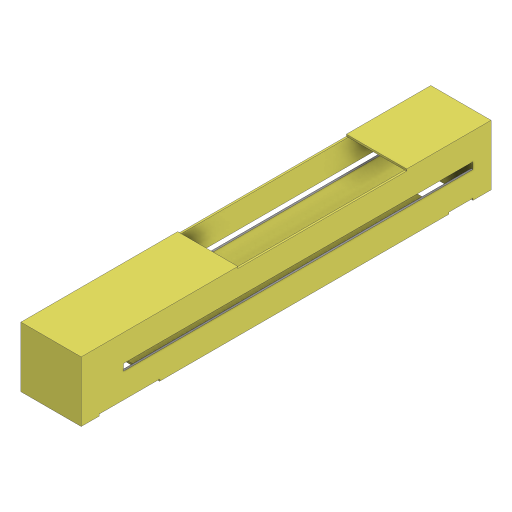
# Autodesk Inventor part: GUIA_CUADRADA
Saved by Autodesk Inventor 2024 (Build 280153000, 153)
## iProperties
Created: 2024-08-15
Part Number: GUIA_CUADRADA
Material: Generic
Document SubType Name: Modeling
Designer: Jhuliams
Density: 1 g/cm^3
Appearance: Default
Author: Jhuliams
Autodesk Inventor part; units mm, degrees
ref_plane "YZ Plane" through (0, 0, 0) normal (1, 0, 0) x (0, 1, 0)
ref_plane "XZ Plane" through (0, 0, 0) normal (0, 1, 0) x (-1, 0, 0)
ref_plane "XY Plane" through (0, 0, 0) normal (0, 0, 1) x (1, 0, 0)
sketch "Sketch1" plane through (0, 0, 0) normal (0, 0, 1) x (1, 0, 0)
  line L0 (-50, 50) -> (50, 50)
  line L1 (50, 50) -> (50, -50)
  line L2 (50, -50) -> (-50, -50)
  line L3 (-50, -50) -> (-50, 50)
  line L4 (-50, 50) -> (50, -50) construction
  line L5 (50, 50) -> (-50, -50) construction
  line L6 (-47, 47) -> (47, 47)
  line L7 (47, 47) -> (47, -47)
  line L8 (47, -47) -> (-47, -47)
  line L9 (-47, -47) -> (-47, 47)
  line L10 (-47, 47) -> (47, -47) construction
  line L11 (47, 47) -> (-47, -47) construction
  point P0 (0, 0)
  dimension "d0" = 100
  dimension "d1" = 100
  dimension "d2" = 94
  dimension "d3" = 94
  constraints: 24 end point, 4 midpoint, 4 parallel, 2 horizontal, 2 perpendicular
  measures "d0" distance of L1.end L2.end
  measures "d1" distance of L0.end L1.end
  measures "d2" distance of L7.end L8.end
  measures "d3" distance of L6.end L7.end
extrude "Extrusion1" add sketch "Sketch1" along normal mid plane 620
sketch "Sketch3" plane through (50, -50, 310) normal (1, 0, 0) x (0, 0, -1)
  line L0 (310, 50) -> (40, 50)
  line L1 (310, 50) -> (620, 50)
  line L2 (620, 50) -> (330, 50)
  line L3 (40, 50) -> (330, 50)
  line L4 (40, 55.5) -> (620, 55.5)
  line L5 (620, 55.5) -> (620, 44.5)
  line L6 (620, 44.5) -> (40, 44.5)
  line L7 (40, 44.5) -> (40, 55.5)
  line L8 (40, 55.5) -> (620, 44.5) construction
  line L9 (620, 55.5) -> (40, 44.5) construction
  dimension "d6" = 270
  dimension "d7" = 310
  dimension "d23" = 290
  dimension "d24" = 580
  dimension "d25" = 11
  constraints: 20 end point, 3 horizontal, 2 midpoint, 2 parallel, 1 collinear, 1 perpendicular, 1 point on line
  measures "d6" distance of L0.start L0.end
  measures "d7" distance of L0.start L1.end
  measures "d23" distance of L0.end L2.end
  measures "d24" distance of L5.end L6.end
  measures "d25" distance of L4.end L5.end
extrude "Extrusion2" cut sketch "Sketch3" against normal blind 620
sketch "Sketch4" plane through (-50, 50, 310) normal (0, 1, 0) x (1, 0, 0)
  line L0 (50, 310) -> (50, 230)
  line L1 (50, 310) -> (50, 510)
  line L2 (50, 510) -> (50, 370)
  line L3 (0, 230) -> (100, 230)
  line L4 (100, 230) -> (100, 510)
  line L5 (100, 510) -> (0, 510)
  line L6 (0, 510) -> (0, 230)
  line L7 (0, 230) -> (100, 510) construction
  line L8 (100, 230) -> (0, 510) construction
  dimension "d12" = 80
  dimension "d13" = 200
  dimension "d14" = 140
  constraints: 18 end point, 2 midpoint, 2 parallel, 2 vertical, 1 horizontal, 1 perpendicular, 1 point on line
  measures "d12" distance of L0.start L0.end
  measures "d13" distance of L0.start L1.end
  measures "d14" distance of L1.end L2.end
extrude "Extrusion3" cut sketch "Sketch4" against normal blind 3
sketch "Sketch5" plane through (-50, -50, 310) normal (0, -1, 0) x (1, 0, 0)
  line L0 (100, -620) -> (100, 0) projected
  line L1 (0, 0) -> (100, 0) projected
  line L2 (0, 0) -> (0, -620) projected
  line L3 (100, -620) -> (0, -620) projected
  line L4 (100, 0) -> (0, 0)
  line L5 (0, 0) -> (0, -100)
  line L6 (0, -100) -> (100, -100)
  line L7 (100, -100) -> (100, 0)
  line L8 (3, -620) -> (3, 0) projected
  line L9 (100, -620) -> (3, -620)
  line L10 (3, -620) -> (3, -580)
  line L11 (3, -580) -> (100, -580)
  line L12 (100, -580) -> (100, -620)
  point P0 (50, -310)
  point P1 (3, -100)
  dimension "d17" = 100
  dimension "d18" = 40
  constraints: 16 end point, 4 parallel, 2 horizontal, 2 perpendicular, 2 point on line
  measures "d17" distance of L5.end L4.end
  measures "d18" distance of L9.end L10.end
sketch "Sketch7" plane through (0, 0, 310) normal (0, 0, 1) x (1, 0, 0)
  line L0 (-50, -50) -> (50, -50) projected
  line L1 (-50, 50) -> (50, 50)
  line L2 (50, 50) -> (50, -50)
  line L3 (50, -50) -> (-50, -50)
  line L4 (-50, -50) -> (-50, 50)
  line L5 (-50, 50) -> (50, -50) construction
  line L6 (50, 50) -> (-50, -50) construction
  point P0 (0, 0)
  constraints: 12 end point, 2 midpoint, 2 parallel, 1 horizontal, 1 perpendicular
extrude "Extrusion4" add sketch "Sketch7" along normal blind 30
extrude "Extrusion5" cut sketch "Sketch5" against normal blind 3 contours L3 L8 L11 L0 | L6 L8 L1 L0
mirror "Mirror1" about plane through (0, 0, 0) normal (0, 0, 1) of "Extrusion4"
body "Solid1"
